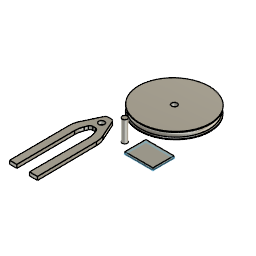
pulley (Autodesk Fusion 360 design; units mm, degrees)
part number: 2025-11-21-09-23-33-273
Autodesk Fusion 360 part; units mm, degrees
sketch "Sketch1" plane through (0, 0, 0) normal (0, 0, 1) x (1, 0, 0)
  line L0 (9.323581, -72.47016) -> (9.388406, -23.373568)
  line L1 (9.388406, -23.373568) -> (19.388397, -23.386771)
  line L2 (19.388397, -23.386771) -> (19.323572, -72.483364)
  line L3 (10.107859, -72.471196) -> (11.168561, -71.252687)
  line L4 (17.030968, -71.067613) -> (18.428639, -72.482182)
  arc A0 (17.030968, -71.067613) -> (11.168561, -71.252687) centre (14.185597, -73.878995) ccw
  line L5 (9.323581, -72.47016) -> (10.107859, -72.471196)
  line L6 (18.428639, -72.482182) -> (19.323572, -72.483364)
  point P0 (14.388401, -23.38017)
  dimension "d8" = 10
  dimension "d35" = 4
  constraint perpendicular L0 L1
  constraint perpendicular L1 L2
  constraint tangent L3 A0
  constraint tangent L4 A0
  constraint perpendicular L0 L5
  constraint perpendicular L2 L6
  measures "d35" radius of A0
revolve "Revolve1" add sketch "Sketch1" angle 360 about axis through (9.388406, -23.373568, 0) along (0.99999913, -0.00132035, 0) contours L0 L1 L2 L3 L4 A0 L5 L6 picked at (14.378457, -38.881025) makes body 1
revolve "Revolve2" add sketch "Sketch1" angle 360 about axis through (9.388406, -23.373568, 0) along (0.99999913, -0.00132035, 0) separate body contours L0 L1 L2 L3 L4 A0 L5 L6 picked at (14.378457, -38.881025) makes body 2
move_body "Move1" bodies 2 to x (0.49867965, -0.49999826, -0.70803979) y (-0.49999826, 0.50132035, -0.70617253) z (0.70803979, 0.70617253, 0) at (5.254655, -7.470353, 0.409671)
hole "Hole1" at (21.54226, -23.792308, 10.147281) direction (0.499339, -0.50066, -0.707107) diameter 4 depth 15 tip angle 180 bodies 2
revolve "Revolve4" add sketch "Sketch1" angle 360 about axis through (9.388406, -23.373568, 0) along (0.99999913, -0.00132035, 0) separate body contours L0 L1 L2 L3 L4 A0 L5 L6 picked at (14.378457, -38.881025) makes body 3
move_body "Move2" bodies 3 1 to x (0.69560549, 0.12170724, -0.70803979) y (-0.69744481, -0.12202905, -0.70617253) z (-0.17234773, 0.98503617, 0) at (-24.978339, -2.195083, -5.003597)
move_body "Move3" bodies 1 3 to x (1, 0, 0) y (0, 1, 0) z (0, 0, 1) at (0, 0, 5)
hole "Hole2" at (-2.435382, 2.24167, 9.645852) direction (0.696526, 0.121868, -0.707107) diameter 5 depth 15 tip angle 180 bodies 1 3
move_face "MoveFace1" to x (1, 0, 0) y (0, 1, 0) z (0, 0, 1) at (0.048411, -0.406784, -0.455195) 1 faces at (-0.024215, 0.172541, 6.950284) on bodies 3
move_face "MoveFace2" to x (1, 0, 0) y (0, 1, 0) z (0, 0, 1) at (0.152045, 0.050682, 0) 1 faces at (2.221993, 0.129165, 4.441358) on bodies 3
sketch "Sketch3" plane through (0, 0, 0) normal (0, 0, 1) x (1, 0, 0)
  line L0 (-41.083167, -3.43352) -> (-52.064909, -26.642468)
  line L1 (-18.083609, -27.862242) -> (-28.984628, -3.510051)
  line L2 (-40.676402, -26.025033) -> (-42.403631, -30.290441)
  line L3 (-27.854076, -30.044738) -> (-29.407007, -26.070549)
  circle A0 centre (-35.000001, -13) radius 4
  line L4 (-54.946668, -39.678122) -> (-54.368527, -124.493951)
  line L5 (-54.368527, -124.493951) -> (-44.032738, -124.423498)
  line L6 (-44.032738, -124.423498) -> (-44.596242, -41.754942)
  line L7 (-25.796642, -41.027866) -> (-25.97631, -124.619625)
  line L8 (-25.97631, -124.619625) -> (-14.469225, -124.644358)
  line L9 (-14.469225, -124.644358) -> (-15.467456, -39.766624)
  arc A1 (-52.064909, -26.642468) -> (-54.946668, -39.678122) centre (-24.947365, -39.473634) ccw
  arc A2 (-42.403631, -30.290441) -> (-44.596242, -41.754942) centre (-14.596939, -41.550454) ccw
  arc A3 (-25.796642, -41.027866) -> (-27.854076, -30.044738) centre (-55.796573, -40.963386) ccw
  arc A4 (-15.467456, -39.766624) -> (-18.083609, -27.862242) centre (-45.465382, -40.119424) ccw
  line L10 (-36.968843, -23.526368) -> (-33.132674, -23.526368)
  line L11 (-37.467494, -1.144342) -> (-32.635531, -1.144342)
  arc A5 (-37.467494, -1.144342) -> (-41.083167, -3.43352) centre (-37.467494, -5.144342) ccw
  arc A6 (-28.984628, -3.510051) -> (-32.635531, -1.144342) centre (-32.635531, -5.144342) ccw
  arc A7 (-36.968843, -23.526368) -> (-40.676402, -26.025033) centre (-36.968843, -27.526368) ccw
  arc A8 (-29.407007, -26.070549) -> (-33.132674, -23.526368) centre (-33.132674, -27.526368) ccw
  dimension "d23" = 8
  dimension "d39" = 30
  dimension "d40" = 30
  dimension "d41" = 30
  dimension "d44" = 4
  dimension "d45" = 4
  constraint perpendicular L4 L5
  constraint perpendicular L5 L6
  constraint perpendicular L7 L8
  constraint tangent L0 A1
  constraint tangent L4 A1
  constraint tangent L2 A2
  constraint tangent L6 A2
  constraint equal A1 A2
  constraint tangent L3 A3
  constraint tangent L7 A3
  constraint tangent L1 A4
  constraint tangent L9 A4
  constraint horizontal L10
  constraint parallel L10 L11
  constraint tangent L11 A5
  constraint tangent L0 A5
  constraint tangent L11 A6
  constraint tangent L1 A6
  constraint equal A5 A6
  constraint tangent L10 A7
  constraint tangent L2 A7
  constraint tangent L10 A8
  constraint tangent L3 A8
  constraint equal A7 A8
  measures "d23" diameter of A0
  measures "d39" radius of A1
  measures "d40" radius of A3
  measures "d41" radius of A4
  measures "d44" radius of A5
  measures "d45" radius of A7
extrude "Extrude1" add sketch "Sketch3" along normal blind 5 separate body contours L0 L1 L2 L3 L4 L5 L6 L7 L8 L9 A1 A2 A3 A4 L10 L11 A5 A6 A7 A8 picked at (-22.080726, -96.763949) makes body 4
sketch "Sketch4" plane through (0, 0, 0) normal (0, 0, 1) x (1, 0, 0)
  circle A0 centre (0, -15) radius 3.75
  dimension "d26" = 7.5
  measures "d26" diameter of A0
extrude "Extrude3" add sketch "Sketch4" along normal blind 30 separate body contours A0 picked at (-1.682513, -15.542355) makes body 5
sketch "Sketch5" plane through (0, 0, 0) normal (0, 0, 1) x (1, 0, 0)
  line L0 (15, 0) -> (55, 0)
  line L1 (55, 0) -> (55, -30)
  line L2 (55, -30) -> (15, -30)
  line L3 (15, -30) -> (15, 0)
  dimension "d31" = 40
  dimension "d32" = 30
  constraint horizontal L0
  constraint vertical L1
  constraint horizontal L2
  constraint vertical L3
  measures "d31" distance of L0.start L0.end
  measures "d32" distance of L0.start L2.end
extrude "Extrude4" add sketch "Sketch5" along normal blind 3 separate body contours L0 L1 L2 L3 picked at (28.333334, -10) makes body 6
move_body "Move4" bodies 3 to x (0.71074264, -0.16179443, -0.68459291) y (0.07381382, 0.98497118, -0.15615152) z (0.69956874, 0.06045113, 0.71200368) at (-7.630026, -2.041727, 6.750622)
move_body "Move5" bodies 3 to x (1, 0, 0) y (0, 1, 0) z (0, 0, 1) at (39.927478, 31.559039, -4.296352)
move_body "Move6" bodies 3 to x (1, 0, 0) y (0, 1, 0) z (0, 0, 1) at (-36.940395, 22.4998, 0.861039)
delete_face "DeleteFace1" 1 faces at (-2.010392, 55.467344, 8.131507) on bodies 3
hole "Hole3" at (0.858813, 54.732807, 11.520021) direction (0.009376, -0.035403, -0.999329) diameter 8 depth 15 tip angle 180 bodies 3
hidden bodies 1 2
